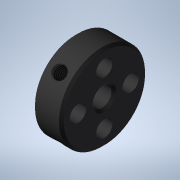
# Autodesk Inventor part: SSCMN4b
Saved by Autodesk Inventor 2024 (Build 280153000, 153)
## iProperties
Category: PARTsolutions
Company: MISUMI
Created: 2025-03-10
Part Number: SSCMN4b
Material: Generic
Catalog Web Link: www.cadenas.de
Description: SCMN, PSCMN, SSCMN_b-Shaft Collars - With Holes
Vendor: MISUMI
Document SubType Name: Modeling
Designer: psAdmin
Manufacturer: MISUMI
Mass: 1.1467 g
Surface Area: 11.3055 cm^2
Volume: 1.1467 cm^3
Density: 1 g/cm^3
Appearance: PSOLRGB-175-175-175
PSOL_IDENT_0: {$CADENAS_DATA/23d-libs/misumi/metric/03_set_collars/scmn/scmn_b.prj},173 {VTYP=3D},{NB=SSCMN4b},{LI
PSOL_IDENT_1: NA=SSCMN4},{NN=SCMN, PSCMN, SSCMN_b},{DATE=02.06.2021 02:59:53},{GEOMDATE=25.12.2015 05:54:25},{VERS
PSOL_IDENT_2: ION=},{LINEID=20},{WBVAR=MAT,ST},{WBNUMERIC=}  {NB=SSCMN4b},{LINA=SSCMN4},{KT=DUMMY},{PN=SSCMN4},{TY
PSOL_IDENT_3: PE=SSCMN},{MAT=304},{ST=-},{AC=Set Screws 2 Pcs. (304 Stainless Steel) },{D=4},{B=6},{D1=18},{S=3.4}
PSOL_IDENT_4: ,{P=11},{M=M3x3},{THMD=3},{THDMIN=2.459},{M1=M3},{M1NDM=3},{C=0.5},{ST0='-','-'},{L=3}
NB: SSCMN4b
NN: SCMN, PSCMN, SSCMN_b
NT: Shaft Collars - With Holes
NBSYN: $PN.b
LINA: SSCMN4
CATALOG: Misumi
PN: SSCMN4
MAT: SUS304 Equivalent
ST: -
AC: Set Screws 2 Pcs. (304 Stainless Steel)
D: 4
B: 6
D1: 18
S: 3.4
P: 11
M: M3x3
M1: M3
SUPPLIER: MISUMI
ARTICLENO: SSCMN4b
BOMINFO: SSCMN4
CREATOR: CADENAS GmbH
Title: SSCMN4
Author: Cadenas PARTsolutions
Comments: Shaft Collars - With Holes
Autodesk Inventor part; units mm, degrees
sketch "Sketch_1" plane through (0, 0, 0) normal (0, 0, 1) x (1, 0, 0)
  line L0 (0, 0) -> (-3, 0)
  line L1 (-3, 2.5) -> (-2.5, 2)
  line L2 (-2.5, 2) -> (2.5, 2)
  line L3 (2.5, 2) -> (3, 2.5)
  line L4 (3, 2.5) -> (3, 8.5)
  line L5 (3, 8.5) -> (2.5, 9)
  line L6 (2.5, 9) -> (-2.5, 9)
  line L7 (-2.5, 9) -> (-3, 8.5)
  line L8 (-3, 8.5) -> (-3, 2.5)
  constraints: 18 end point
revolve "Revolution1" add sketch "Sketch_1" angle 360 about axis through (0, 0, 0) along (1, 0, 0)
sketch "Sketch_2" plane through (0, 0, 0) normal (1, 0, 0) x (0, 1, 0)
  line L0 (7.0004, 7.0004) -> (0.7778, 0.7778)
  line L1 (0.7778, 0.7778) -> (-0.2828, 1.8385)
  line L2 (-0.2828, 1.8385) -> (0.3536, 2.4749)
  line L3 (0.3536, 2.4749) -> (0.7361, 2.4749)
  line L4 (0.7361, 2.4749) -> (5.3033, 7.0421)
  line L5 (5.3033, 7.0421) -> (5.3033, 7.4246)
  line L6 (5.3033, 7.4246) -> (5.9397, 8.061)
  line L7 (5.9397, 8.061) -> (7.0004, 7.0004)
  line L8 (7.0004, 7.0004) -> (0.7778, 0.7778)
  constraints: 18 end point
revolve "Revolution2" cut sketch "Sketch_2" angle 360 about axis through (0, 7.0004, 7.0004) along (0, 0.7071068, 0.7071068)
thread "Thread1" size "M3x0.5" class "6H" standard "ISO Metric profile" full length
sketch "Sketch_3" plane through (0, 0, 0) normal (1, 0, 0) x (0, 1, 0)
  line L0 (-7.0004, 7.0004) -> (-0.7778, 0.7778)
  line L1 (-0.7778, 0.7778) -> (-1.8385, -0.2828)
  line L2 (-1.8385, -0.2828) -> (-2.4749, 0.3536)
  line L3 (-2.4749, 0.3536) -> (-2.4749, 0.7361)
  line L4 (-2.4749, 0.7361) -> (-7.0421, 5.3033)
  line L5 (-7.0421, 5.3033) -> (-7.4246, 5.3033)
  line L6 (-7.4246, 5.3033) -> (-8.061, 5.9397)
  line L7 (-8.061, 5.9397) -> (-7.0004, 7.0004)
  line L8 (-7.0004, 7.0004) -> (-0.7778, 0.7778)
  constraints: 18 end point
revolve "Revolution3" cut sketch "Sketch_3" angle 360 about axis through (0, -7.0004, 7.0004) along (0, -0.7071068, 0.7071068)
thread "Thread2" size "M3x0.5" class "6H" standard "ISO Metric profile" full length
sketch "Sketch_6" plane through (0, 0, 0) normal (1, 0, 0) x (0, 1, 0)
  circle A0 centre (0, -5.5) radius 1.7
  constraints: 1 centre point
extrude "Extrusion1" cut sketch "Sketch_6" along normal mid plane 12
sketch "Sketch_7" plane through (0, 0, 0) normal (1, 0, 0) x (0, 1, 0)
  circle A0 centre (0, 5.5) radius 1.7
  constraints: 1 centre point
extrude "Extrusion2" cut sketch "Sketch_7" along normal mid plane 12
sketch "Sketch_5" plane through (0, 0, 0) normal (1, 0, 0) x (0, 1, 0)
  circle A0 centre (5.5, 0) radius 1.7
  constraints: 1 centre point
extrude "Extrusion3" cut sketch "Sketch_5" along normal mid plane 6
sketch "Sketch_9" plane through (0, 0, 0) normal (1, 0, 0) x (0, 1, 0)
  circle A0 centre (-5.5, 0) radius 1.7
  constraints: 1 centre point
extrude "Extrusion4" cut sketch "Sketch_9" along normal mid plane 6
ref_plane "body_set_h_XY" through (0, -6.364, 6.364) normal (0, 0.7071068, -0.7071068) x (1, 0, 0)
ref_plane "body_set_h_YZ" through (0, -6.364, 6.364) normal (1, 0, 0) x (0, -0.7071068, -0.7071068)
ref_plane "body_set_h_ZX" through (0, -6.364, 6.364) normal (0, -0.7071068, -0.7071068) x (0, 0.7071068, -0.7071068)
ref_plane "body_set_v_XY" through (0, 6.364, 6.364) normal (0, 0.7071068, 0.7071068) x (1, 0, 0)
ref_plane "body_set_v_YZ" through (0, 6.364, 6.364) normal (1, 0, 0) x (0, 0.7071068, -0.7071068)
ref_plane "body_set_v_ZX" through (0, 6.364, 6.364) normal (0, 0.7071068, -0.7071068) x (0, 0.7071068, 0.7071068)
body "Solid1"
